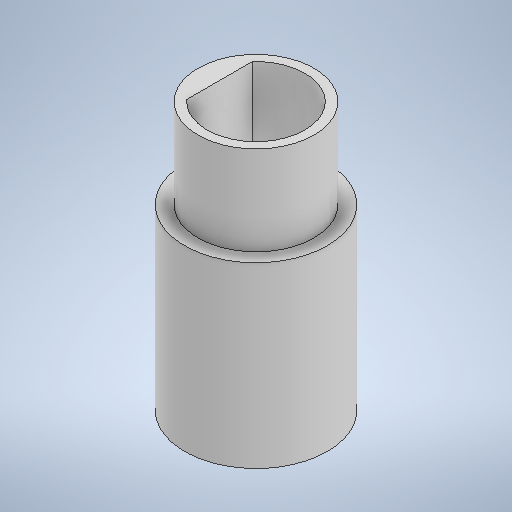
# Autodesk Inventor part: 5.5x4.8
Saved by Autodesk Inventor 2025 (Build 290162010, 162A)
## iProperties
Created: 2025-03-23
Part Number: 5.5x4.8
Material: Generic
Document SubType Name: Modeling
Designer: aduwa
Density: 1 g/cm^3
Appearance: Default
Author: aduwa
Autodesk Inventor part; units mm, degrees
ref_plane "YZ Plane" through (0, 0, 0) normal (1, 0, 0) x (0, 1, 0)
ref_plane "XZ Plane" through (0, 0, 0) normal (0, 1, 0) x (-1, 0, 0)
ref_plane "XY Plane" through (0, 0, 0) normal (0, 0, 1) x (1, 0, 0)
sketch "Sketch1" plane through (0, 0, 0) normal (0, 1, 0) x (-1, 0, 0)
  arc A0 (2.05, 1.833) -> (2.05, -1.833) centre (0, 0) ccw
  line L0 (-2.75, 2.2253) -> (-2.75, -2.0609)
  circle A1 centre (0, 0) radius 4
  line L1 (2.05, 1.833) -> (2.05, -1.833)
  dimension "d0" = 5.5
  dimension "d3" = 8
  dimension "d4" = 4.8
  constraints: 4 end point, 2 centre point, 2 coincident, 2 point on circle, 2 vertical, 1 tangent
  measures "d0" diameter of A0
  measures "d3" diameter of A1
  measures "d4" distance between parallel lines of L1 L0
extrude "Extrusion1" add sketch "Sketch1" along normal blind 15
sketch "Sketch2" plane through (0, 15, 0) normal (0, 1, 0) x (1, 0, 0)
  circle A0 centre (0, 0) radius 3.25
  circle A1 centre (0, 0) radius 4 projected
  dimension "d7" = 6.5
  constraints: 1 centre point, 1 coincident
  measures "d7" diameter of A0
extrude "Extrusion2" cut sketch "Sketch2" against normal blind 5
body "Solid1"
